Autodesk Inventor part; units mm, degrees
(part 5 of 5)
  arc A2073 (17.0347, 6.1889) -> (16.978, 6.1961) centre (16.9429, 5.6908) ccw
  arc A2074 (17.0769, 6.1787) -> (17.0347, 6.1889) centre (16.9634, 5.8019) ccw
  arc A2075 (17.0863, 6.166) -> (17.0769, 6.1787) centre (17.0731, 6.166) ccw
  arc A2076 (17.0803, 6.1441) -> (17.0863, 6.166) centre (17.0434, 6.166) ccw
  arc A2077 (17.0246, 6.0516) -> (17.0803, 6.1441) centre (9.6636, 10.5426) ccw
  arc A2078 (16.9568, 5.9437) -> (17.0246, 6.0516) centre (12.9822, 8.5179) ccw
  arc A2079 (16.8763, 5.8218) -> (16.9568, 5.9437) centre (10.125, 10.3684) ccw
  arc A2080 (16.8763, 5.8218) -> (16.7706, 5.6513) centre (19.0678, 4.346) ccw
  arc A2081 (16.7706, 5.6513) -> (16.7087, 5.5153) centre (17.4985, 5.2377) ccw
  arc A2082 (16.7087, 5.5153) -> (16.6768, 5.3823) centre (17.3385, 5.2939) ccw
  arc A2083 (16.6768, 5.3823) -> (16.6663, 5.2242) centre (17.8608, 5.2242) ccw
  line L590 (16.6663, 5.2242) -> (16.6663, 4.9384)
  line L591 (16.6663, 4.9384) -> (16.8763, 4.9384)
  arc A2084 (17.0024, 4.933) -> (16.8763, 4.9384) centre (16.8763, 3.4518) ccw
  arc A2085 (17.055, 4.9096) -> (17.0024, 4.933) centre (16.995, 4.8457) ccw
  arc A2086 (17.0794, 4.8597) -> (17.055, 4.9096) centre (17.0013, 4.8525) ccw
  arc A2087 (17.0842, 4.7434) -> (17.0794, 4.8597) centre (15.9599, 4.7557) ccw
  arc A2088 (17.0818, 4.6144) -> (17.0842, 4.7434) centre (8.0084, 4.8424) ccw
  arc A2089 (17.0719, 4.5944) -> (17.0818, 4.6144) centre (17.0553, 4.6151) ccw
  arc A2090 (17.0566, 4.5972) -> (17.0719, 4.5944) centre (17.0655, 4.6024) ccw
  arc A2091 (17.0078, 4.682) -> (17.0566, 4.5972) centre (19.8706, 6.2728) ccw
  line L592 (17.0078, 4.682) -> (16.9335, 4.8157)
  line L593 (16.9335, 4.8157) -> (16.7399, 4.6979)
  line L594 (16.7399, 4.6979) -> (16.5463, 4.5802)
  line L595 (16.5463, 4.5802) -> (16.5463, 5.2473)
  arc A2092 (16.5624, 5.6854) -> (16.5463, 5.2473) centre (22.4968, 5.2473) ccw
  arc A2093 (16.6109, 6.1015) -> (16.5624, 5.6854) centre (21.5063, 5.3204) ccw
  arc A2094 (16.6672, 6.3078) -> (16.6109, 6.1015) centre (17.5877, 5.9456) ccw
  arc A2095 (16.7148, 6.3034) -> (16.6672, 6.3078) centre (16.6904, 6.2987) ccw
  arc A2096 (16.7148, 6.3034) -> (16.735, 6.2571) centre (16.8277, 6.3252) ccw
  arc A2097 (16.735, 6.2571) -> (16.7731, 6.2241) centre (16.8271, 6.3248) ccw
  arc A2098 (16.7731, 6.2241) -> (16.8311, 6.2046) centre (16.8596, 6.3854) ccw
  arc A2099 (16.8311, 6.2046) -> (16.9107, 6.1984) centre (16.9107, 6.7106) ccw
  arc A2100 (18.2103, 6.1151) -> (18.2263, 6.1384) centre (18.2013, 6.1384) ccw
  arc A2101 (18.147, 6.096) -> (18.2103, 6.1151) centre (18.0499, 6.533) ccw
  arc A2102 (18.0598, 6.0827) -> (18.147, 6.096) centre (18.005, 6.7348) ccw
  arc A2103 (17.9563, 6.0784) -> (18.0598, 6.0827) centre (17.9563, 7.3152) ccw
  arc A2104 (17.8528, 6.0827) -> (17.9563, 6.0784) centre (17.9563, 7.3152) ccw
  arc A2105 (17.7656, 6.096) -> (17.8528, 6.0827) centre (17.9075, 6.7348) ccw
  arc A2106 (17.7023, 6.1151) -> (17.7656, 6.096) centre (17.8627, 6.533) ccw
  arc A2107 (17.6863, 6.1384) -> (17.7023, 6.1151) centre (17.7112, 6.1384) ccw
  arc A2108 (17.7023, 6.1617) -> (17.6863, 6.1384) centre (17.7112, 6.1384) ccw
  arc A2109 (17.7656, 6.1808) -> (17.7023, 6.1617) centre (17.8627, 5.7438) ccw
  arc A2110 (17.8528, 6.1941) -> (17.7656, 6.1808) centre (17.9075, 5.542) ccw
  arc A2111 (17.9563, 6.1984) -> (17.8528, 6.1941) centre (17.9563, 4.9616) ccw
  arc A2112 (18.0598, 6.1941) -> (17.9563, 6.1984) centre (17.9563, 4.9616) ccw
  arc A2113 (18.147, 6.1808) -> (18.0598, 6.1941) centre (18.005, 5.542) ccw
  arc A2114 (18.2103, 6.1617) -> (18.147, 6.1808) centre (18.0499, 5.7438) ccw
  arc A2115 (18.2263, 6.1384) -> (18.2103, 6.1617) centre (18.2013, 6.1384) ccw
  arc A2116 (18.9393, 6.1155) -> (18.9463, 6.1384) centre (18.9051, 6.1384) ccw
  arc A2117 (18.9198, 6.096) -> (18.9393, 6.1155) centre (18.8808, 6.1546) ccw
  arc A2118 (18.8907, 6.0829) -> (18.9198, 6.096) centre (18.8657, 6.1773) ccw
  arc A2119 (18.8563, 6.0784) -> (18.8907, 6.0829) centre (18.8563, 6.2127) ccw
  arc A2120 (18.8219, 6.0829) -> (18.8563, 6.0784) centre (18.8563, 6.2127) ccw
  arc A2121 (18.7927, 6.096) -> (18.8219, 6.0829) centre (18.8469, 6.1773) ccw
  arc A2122 (18.7732, 6.1155) -> (18.7927, 6.096) centre (18.8318, 6.1546) ccw
  arc A2123 (18.7663, 6.1384) -> (18.7732, 6.1155) centre (18.8075, 6.1384) ccw
  arc A2124 (18.7732, 6.1613) -> (18.7663, 6.1384) centre (18.8075, 6.1384) ccw
  arc A2125 (18.7927, 6.1808) -> (18.7732, 6.1613) centre (18.8318, 6.1222) ccw
  arc A2126 (18.8219, 6.1939) -> (18.7927, 6.1808) centre (18.8469, 6.0995) ccw
  arc A2127 (18.8563, 6.1984) -> (18.8219, 6.1939) centre (18.8563, 6.0641) ccw
  arc A2128 (18.8907, 6.1939) -> (18.8563, 6.1984) centre (18.8563, 6.0641) ccw
  arc A2129 (18.9198, 6.1808) -> (18.8907, 6.1939) centre (18.8657, 6.0995) ccw
  arc A2130 (18.9393, 6.1613) -> (18.9198, 6.1808) centre (18.8808, 6.1222) ccw
  arc A2131 (18.9463, 6.1384) -> (18.9393, 6.1613) centre (18.9051, 6.1384) ccw
  arc A2132 (18.0251, 5.5941) -> (17.9001, 5.5984) centre (17.9001, 3.7904) ccw
  arc A2133 (18.1305, 5.5808) -> (18.0251, 5.5941) centre (17.9599, 4.6537) ccw
  arc A2134 (18.2088, 5.5619) -> (18.1305, 5.5808) centre (17.9977, 4.8593) ccw
  arc A2135 (18.2263, 5.5384) -> (18.2088, 5.5619) centre (18.2018, 5.5384) ccw
  arc A2136 (18.2112, 5.5152) -> (18.2263, 5.5384) centre (18.2008, 5.5384) ccw
  arc A2137 (18.1558, 5.496) -> (18.2112, 5.5152) centre (18.0745, 5.8213) ccw
  arc A2138 (18.0783, 5.4827) -> (18.1558, 5.496) centre (18.029, 6.0032) ccw
  arc A2139 (17.9863, 5.4784) -> (18.0783, 5.4827) centre (17.9863, 6.4544) ccw
  line L596 (17.9863, 5.4784) -> (17.7463, 5.4784)
  line L597 (17.7463, 5.4784) -> (17.7463, 5.2384)
  line L598 (17.7463, 5.2384) -> (17.7463, 4.9984)
  line L599 (17.7463, 4.9984) -> (17.9863, 4.9984)
  arc A2140 (18.0783, 4.9941) -> (17.9863, 4.9984) centre (17.9863, 4.0224) ccw
  arc A2141 (18.1558, 4.9808) -> (18.0783, 4.9941) centre (18.029, 4.4736) ccw
  arc A2142 (18.2112, 4.9616) -> (18.1558, 4.9808) centre (18.0745, 4.6555) ccw
  arc A2143 (18.2263, 4.9384) -> (18.2112, 4.9616) centre (18.2008, 4.9384) ccw
  arc A2144 (18.2103, 4.9151) -> (18.2263, 4.9384) centre (18.2013, 4.9384) ccw
  arc A2145 (18.147, 4.896) -> (18.2103, 4.9151) centre (18.0499, 5.333) ccw
  arc A2146 (18.0598, 4.8827) -> (18.147, 4.896) centre (18.005, 5.5348) ccw
  arc A2147 (17.9563, 4.8784) -> (18.0598, 4.8827) centre (17.9563, 6.1152) ccw
  arc A2148 (17.9563, 4.8784) -> (17.7812, 4.8742) centre (17.9563, 1.2357) ccw
  arc A2149 (17.7812, 4.8742) -> (17.7206, 4.8517) centre (17.7864, 4.7671) ccw
  arc A2150 (17.7206, 4.8517) -> (17.6926, 4.801) centre (17.7655, 4.7939) ccw
  arc A2151 (17.6926, 4.801) -> (17.6863, 4.6684) centre (19.0709, 4.6684) ccw
  arc A2152 (17.6863, 4.6684) -> (17.6926, 4.5358) centre (19.0709, 4.6684) ccw
  arc A2153 (17.6926, 4.5358) -> (17.7206, 4.4851) centre (17.7655, 4.5429) ccw
  arc A2154 (17.7206, 4.4851) -> (17.7812, 4.4626) centre (17.7864, 4.5697) ccw
  arc A2155 (17.7812, 4.4626) -> (17.9563, 4.4584) centre (17.9563, 8.1011) ccw
  arc A2156 (18.0598, 4.4541) -> (17.9563, 4.4584) centre (17.9563, 3.2216) ccw
  arc A2157 (18.147, 4.4408) -> (18.0598, 4.4541) centre (18.005, 3.802) ccw
  arc A2158 (18.2103, 4.4217) -> (18.147, 4.4408) centre (18.0499, 4.0038) ccw
  arc A2159 (18.2263, 4.3984) -> (18.2103, 4.4217) centre (18.2013, 4.3984) ccw
  arc A2160 (18.2089, 4.375) -> (18.2263, 4.3984) centre (18.2018, 4.3984) ccw
  arc A2161 (18.1318, 4.356) -> (18.2089, 4.375) centre (18.0023, 5.0504) ccw
  arc A2162 (18.0279, 4.3427) -> (18.1318, 4.356) centre (17.9636, 5.2577) ccw
  arc A2163 (17.9046, 4.3384) -> (18.0279, 4.3427) centre (17.9046, 6.096) ccw
  line L600 (17.9046, 4.3384) -> (17.583, 4.3384)
  line L601 (17.583, 4.3384) -> (17.6128, 4.9084)
  line L602 (17.6128, 4.9084) -> (17.6426, 5.4784)
  line L603 (17.6426, 5.4784) -> (17.4545, 5.4784)
  arc A2164 (17.3823, 5.4806) -> (17.4545, 5.4784) centre (17.4545, 6.6497) ccw
  arc A2165 (17.3216, 5.4875) -> (17.3823, 5.4806) centre (17.4197, 6.0862) ccw
  arc A2166 (17.2756, 5.4971) -> (17.3216, 5.4875) centre (17.4052, 5.9979) ccw
  arc A2167 (17.2663, 5.5092) -> (17.2756, 5.4971) centre (17.2788, 5.5092) ccw
  arc A2168 (17.2713, 5.5292) -> (17.2663, 5.5092) centre (17.3085, 5.5092) ccw
  arc A2169 (17.3059, 5.5919) -> (17.2713, 5.5292) centre (20.1068, 4.0042) ccw
  arc A2170 (17.3496, 5.6657) -> (17.3059, 5.5919) centre (19.3657, 4.4243) ccw
  arc A2171 (17.4013, 5.7474) -> (17.3496, 5.6657) centre (20.6021, 3.663) ccw
  line L604 (17.4013, 5.7474) -> (17.5363, 5.9547)
  line L605 (17.5363, 5.9547) -> (17.5551, 5.7765)
  arc A2172 (17.5551, 5.7765) -> (17.5761, 5.6701) centre (18.156, 5.84) ccw
  arc A2173 (17.5761, 5.6701) -> (17.6154, 5.6225) centre (17.6514, 5.6921) ccw
  arc A2174 (17.6154, 5.6225) -> (17.6924, 5.6022) centre (17.6992, 5.7847) ccw
  arc A2175 (17.6924, 5.6022) -> (17.9001, 5.5984) centre (17.9001, 11.2336) ccw
  arc A2176 (18.9393, 5.5155) -> (18.9463, 5.5384) centre (18.9051, 5.5384) ccw
  arc A2177 (18.9198, 5.496) -> (18.9393, 5.5155) centre (18.8808, 5.5546) ccw
  arc A2178 (18.8907, 5.4829) -> (18.9198, 5.496) centre (18.8657, 5.5773) ccw
  arc A2179 (18.8563, 5.4784) -> (18.8907, 5.4829) centre (18.8563, 5.6127) ccw
  arc A2180 (18.8219, 5.4829) -> (18.8563, 5.4784) centre (18.8563, 5.6127) ccw
  arc A2181 (18.7927, 5.496) -> (18.8219, 5.4829) centre (18.8469, 5.5773) ccw
  arc A2182 (18.7732, 5.5155) -> (18.7927, 5.496) centre (18.8318, 5.5546) ccw
  arc A2183 (18.7663, 5.5384) -> (18.7732, 5.5155) centre (18.8075, 5.5384) ccw
  arc A2184 (18.7732, 5.5613) -> (18.7663, 5.5384) centre (18.8075, 5.5384) ccw
  arc A2185 (18.7927, 5.5808) -> (18.7732, 5.5613) centre (18.8318, 5.5222) ccw
  arc A2186 (18.8219, 5.5939) -> (18.7927, 5.5808) centre (18.8469, 5.4995) ccw
  arc A2187 (18.8563, 5.5984) -> (18.8219, 5.5939) centre (18.8563, 5.4641) ccw
  arc A2188 (18.8907, 5.5939) -> (18.8563, 5.5984) centre (18.8563, 5.4641) ccw
  arc A2189 (18.9198, 5.5808) -> (18.8907, 5.5939) centre (18.8657, 5.4995) ccw
  arc A2190 (18.9393, 5.5613) -> (18.9198, 5.5808) centre (18.8808, 5.5222) ccw
  arc A2191 (18.9463, 5.5384) -> (18.9393, 5.5613) centre (18.9051, 5.5384) ccw
  arc A2192 (18.098, 3.9148) -> (17.9003, 3.9184) centre (17.9003, -1.5446) ccw
  arc A2193 (18.1769, 3.8969) -> (18.098, 3.9148) centre (18.0901, 3.698) ccw
  arc A2194 (18.2139, 3.8558) -> (18.1769, 3.8969) centre (18.1501, 3.8355) ccw
  arc A2195 (18.2263, 3.7761) -> (18.2139, 3.8558) centre (17.9637, 3.7761) ccw
  arc A2196 (18.2174, 3.6941) -> (18.2263, 3.7761) centre (17.8442, 3.7761) ccw
  arc A2197 (18.1872, 3.661) -> (18.2174, 3.6941) centre (18.1735, 3.7037) ccw
  arc A2198 (18.1238, 3.656) -> (18.1872, 3.661) centre (18.1449, 3.7931) ccw
  arc A2199 (17.9459, 3.6863) -> (18.1238, 3.656) centre (18.9762, 9.2014) ccw
  arc A2200 (17.7129, 3.747) -> (17.9459, 3.6863) centre (18.2599, 5.3673) ccw
  arc A2201 (17.5691, 3.8307) -> (17.7129, 3.747) centre (17.846, 4.1411) ccw
  arc A2202 (17.5014, 3.9422) -> (17.5691, 3.8307) centre (17.7176, 3.9971) ccw
  arc A2203 (17.4989, 4.0849) -> (17.5014, 3.9422) centre (17.8035, 4.0189) ccw
  line L606 (17.4989, 4.0849) -> (17.5343, 4.2484)
  line L607 (17.5343, 4.2484) -> (17.5543, 4.0834)
  arc A2204 (17.5543, 4.0834) -> (17.5768, 3.9875) centre (17.9997, 4.1373) ccw
  arc A2205 (17.5768, 3.9875) -> (17.6179, 3.9419) centre (17.6524, 4.0143) ccw
  arc A2206 (17.6179, 3.9419) -> (17.6975, 3.9223) centre (17.7053, 4.1252) ccw
  arc A2207 (17.6975, 3.9223) -> (17.9003, 3.9184) centre (17.9003, 9.2161) ccw
  line L608 (0, 24) -> (0, 0)
  line L609 (0, 24) -> (68, 24)
  line L610 (0, 0) -> (68, 0)
  line L611 (68, 0) -> (68, 24)
  point P0 (12.7063, 20.8384)
  point P1 (11.8063, 20.0584)
  point P2 (11.9213, 20.0541)
  point P3 (12.0182, 20.0408)
  point P4 (12.0894, 20.0218)
  point P5 (12.0881, 19.9747)
  point P6 (12.0013, 19.9559)
  point P7 (11.8853, 19.9427)
  point P8 (11.7463, 19.9384)
  point P9 (12.1159, 19.2586)
  point P10 (12.0459, 19.1953)
  point P11 (11.9397, 19.1189)
  point P12 (11.8188, 19.0431)
  point P13 (11.7004, 18.9795)
  point P14 (11.5903, 18.9251)
  point P15 (11.4946, 18.8771)
  point P16 (11.4126, 18.8354)
  point P17 (11.3986, 18.8266)
  point P18 (11.3934, 18.8135)
  point P19 (11.4069, 18.7341)
  point P20 (11.426, 18.64)
  point P21 (11.4519, 18.5309)
  point P22 (11.4937, 18.3833)
  point P23 (11.5309, 18.3093)
  point P24 (11.5753, 18.2784)
  point P25 (11.6346, 18.278)
  point P26 (11.6941, 18.2678)
  point P27 (11.7291, 18.2158)
  point P28 (11.7436, 18.0852)
  point P29 (11.7463, 17.7428)
  point P30 (12.0463, 17.1784)
  point P31 (12.2148, 17.1823)
  point P32 (12.2938, 17.1994)
  point P33 (12.3322, 17.2356)
  point P34 (12.3463, 17.2984)
  point P35 (12.425, 17.3999)
  point P36 (12.5482, 17.4154)
  point P37 (12.8563, 17.4184)
  point P38 (13.087, 19.1584)
  point P39 (12.9007, 19.1601)
  point P40 (12.8581, 19.174)
  point P41 (12.8536, 19.2022)
  point P42 (12.9163, 19.2784)
  point P43 (12.9789, 19.3313)
  point P44 (13.0561, 19.3688)
  point P45 (13.1494, 19.3911)
  point P46 (13.26, 19.3984)
  point P47 (13.4792, 19.6989)
  point P48 (13.478, 19.8229)
  point P49 (13.4881, 19.9345)
  point P50 (13.5071, 20.0236)
  point P51 (13.5348, 20.0709)
  point P52 (13.5721, 20.0577)
  point P53 (13.5913, 19.8102)
  point P54 (13.6033, 19.3928)
  point P55 (13.6063, 18.6304)
  point P56 (14.5932, 20.0139)
  point P57 (14.5548, 19.8888)
  point P58 (14.5113, 19.7473)
  point P59 (14.4699, 19.6124)
  point P60 (14.4378, 19.5078)
  point P61 (14.4081, 19.3727)
  point P62 (14.4088, 19.2573)
  point P63 (14.4428, 19.1194)
  point P64 (14.5281, 18.8922)
  point P65 (14.6638, 18.5071)
  point P66 (14.6749, 18.2941)
  point P67 (14.5827, 18.1798)
  point P68 (14.3814, 18.1384)
  point P69 (14.3039, 18.126)
  point P70 (14.2749, 18.0893)
  point P71 (14.2823, 18.0105)
  point P72 (14.35, 17.7784)
  point P73 (14.4059, 17.613)
  point P74 (14.4515, 17.5474)
  point P75 (14.5184, 17.5192)
  point P76 (14.6535, 17.5156)
  point P77 (14.9602, 17.5767)
  point P78 (15.1627, 17.7314)
  point P79 (15.265, 17.9912)
  point P80 (15.2712, 18.3686)
  point P81 (15.2496, 18.5236)
  point P82 (15.21, 18.7037)
  point P83 (15.1602, 18.8801)
  point P84 (15.107, 19.0234)
  point P85 (13.6063, 20.7484)
  point P86 (13.5986, 20.6416)
  point P87 (13.5679, 20.6062)
  point P88 (13.5164, 20.6153)
  point P89 (13.4203, 20.6938)
  point P90 (13.3559, 20.7423)
  point P91 (13.3148, 20.7442)
  point P92 (13.2758, 20.7081)
  point P93 (13.2086, 20.5888)
  point P94 (13.1538, 20.4911)
  point P95 (13.1203, 20.454)
  point P96 (13.097, 20.457)
  point P97 (13.0799, 20.4934)
  point P98 (13.0197, 20.5725)
  point P99 (12.9611, 20.5921)
  point P100 (12.8819, 20.5984)
  point P101 (12.7788, 20.6059)
  point P102 (12.7323, 20.6339)
  point P103 (12.7109, 20.693)
  point P104 (12.7556, 17.8982)
  point P105 (12.725, 17.862)
  point P106 (12.6657, 17.8433)
  point P107 (12.4468, 17.8433)
  point P108 (12.3875, 17.862)
  point P109 (12.3569, 17.8982)
  point P110 (12.3463, 17.9584)
  point P111 (12.3569, 18.0185)
  point P112 (12.3875, 18.0548)
  point P113 (12.4468, 18.0735)
  point P114 (12.5563, 18.0784)
  point P115 (12.6657, 18.0735)
  point P116 (12.725, 18.0548)
  point P117 (12.7556, 18.0185)
  point P118 (12.7556, 18.5582)
  point P119 (12.725, 18.522)
  point P120 (12.6657, 18.5033)
  point P121 (12.4468, 18.5033)
  point P122 (12.3875, 18.522)
  point P123 (12.3569, 18.5582)
  point P124 (12.3569, 18.6785)
  point P125 (12.3875, 18.7148)
  point P126 (12.4468, 18.7335)
  point P127 (12.5563, 18.7384)
  point P128 (12.6657, 18.7335)
  point P129 (12.725, 18.7148)
  point P130 (12.7556, 18.6785)
  point P131 (12.7663, 18.6184)
  point P132 (12.7663, 19.9384)
  point P133 (12.7434, 19.943)
  point P134 (12.8217, 20.0213)
  point P135 (10.2183, 18.1693)
  point P136 (10.0906, 18.2722)
  point P137 (9.9804, 18.3585)
  point P138 (9.8833, 18.4328)
  point P139 (9.8721, 18.4355)
  point P140 (9.8612, 18.431)
  point P141 (9.8035, 18.3927)
  point P142 (9.7368, 18.3474)
  point P143 (9.6607, 18.2942)
  point P144 (9.5952, 17.9907)
  point P145 (9.6704, 17.9062)
  point P146 (9.8031, 17.7781)
  point P147 (9.9578, 17.6378)
  point P148 (10.1207, 17.499)
  point P149 (10.6542, 17.3404)
  point P150 (10.8211, 17.5537)
  point P151 (10.8643, 17.6563)
  point P152 (10.8379, 17.7313)
  point P153 (10.7285, 17.8072)
  point P154 (10.6375, 17.8607)
  point P155 (10.5045, 17.9519)
  point P156 (10.358, 18.0595)
  point P157 (7.3271, 17.7998)
  point P158 (7.1576, 17.6869)
  point P159 (7.1147, 17.6052)
  point P160 (7.1453, 17.5068)
  point P161 (7.307, 17.3046)
  point P162 (7.3807, 17.2275)
  point P163 (7.4351, 17.1973)
  point P164 (7.4946, 17.1979)
  point P165 (7.5838, 17.2309)
  point P166 (7.7872, 17.3447)
  point P167 (7.9869, 17.499)
  point P168 (8.1701, 17.6827)
  point P169 (8.3244, 17.8844)
  point P170 (8.3941, 17.9924)
  point P171 (8.4528, 18.0896)
  point P172 (8.4998, 18.1724)
  point P173 (8.4823, 18.2379)
  point P174 (8.2984, 18.3345)
  point P175 (8.1156, 18.4216)
  point P176 (8.0392, 18.4333)
  point P177 (8.014, 18.4217)
  point P178 (7.9487, 18.3598)
  point P179 (7.873, 18.2817)
  point P180 (7.7913, 18.19)
  point P181 (7.6941, 18.0877)
  point P182 (7.5704, 17.9771)
  point P183 (7.4412, 17.8752)
  point P184 (8.4343, 17.6584)
  point P185 (8.3104, 17.6526)
  point P186 (8.2783, 17.6247)
  point P187 (8.2818, 17.5682)
  point P188 (8.3628, 17.3596)
  point P189 (8.43, 17.2112)
  point P190 (8.4859, 17.1505)
  point P191 (8.5685, 17.1243)
  point P192 (8.7555, 17.1184)
  point P193 (8.9113, 17.1254)
  point P194 (9.0215, 17.1483)
  point P195 (9.1109, 17.1926)
  point P196 (9.199, 17.2657)
  point P197 (9.2804, 17.3685)
  point P198 (9.3231, 17.4751)
  point P199 (9.3419, 17.6329)
  constraints: 4416 point on circle, 2208 centre point, 1224 end point
extrude "押し出し3" cut sketch "スケッチ3" against normal blind 5 contours L609 L611 L610 L608
equation "\"d1\" = d0"
equation "\"d2\" = d1"
equation "\"d3\" = d0"
